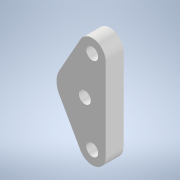
# Autodesk Inventor part: belt_tender_2
Saved by Autodesk Inventor 2020 (Build 240168000, 168)
## iProperties
Created: 2019-09-03
Part Number: belt_tender_2
Material: Generic
Document SubType Name: Modeling
Designer: psrob
Density: 1 g/cm^3
Appearance: Default
Author: psrob
Autodesk Inventor part; units mm, degrees
ref_plane "YZ Plane" through (0, 0, 0) normal (1, 0, 0) x (0, 1, 0)
ref_plane "XZ Plane" through (0, 0, 0) normal (0, 1, 0) x (-1, 0, 0)
ref_plane "XY Plane" through (0, 0, 0) normal (0, 0, 1) x (1, 0, 0)
sketch "Sketch1" plane through (0, 0, 0) normal (0, 0, 1) x (1, 0, 0)
  line L0 (0.625, 2.5) -> (2.625, 2.5) projected
  line L1 (4.125, 1) -> (2.625, 2.5) projected
  line L2 (4.125, 7) -> (4.125, 1) projected
  arc A0 (4.125, 7) -> (-0.0865, 8.1023) centre (1.875, 7) ccw projected
  line L3 (-3.6762, 1.7147) -> (-0.0865, 8.1023) projected
  arc A1 (-3.6762, 1.7147) -> (-3.6762, -1.7147) centre (-0.625, 0) ccw projected
  line L4 (-0.0865, -8.1023) -> (-3.6762, -1.7147) projected
  arc A2 (-0.0865, -8.1023) -> (4.125, -7) centre (1.875, -7) ccw projected
  line L5 (4.125, -1) -> (4.125, -7) projected
  line L6 (2.625, -2.5) -> (4.125, -1) projected
  line L7 (2.625, -2.5) -> (0.625, -2.5) projected
  arc A3 (0.625, 2.5) -> (0.625, -2.5) centre (0.625, 0) ccw projected
  circle A4 centre (1.875, 7) radius 1 projected
  circle A5 centre (1.875, -7) radius 1 projected
  circle A6 centre (0.625, 0) radius 1 projected
  line L8 (4.125, -1) -> (2.625, -2.5) projected
  line L9 (4.125, 1) -> (4.125, -1) projected
  line L10 (2.625, 2.5) -> (4.125, 1) projected
  line L11 (2.625, 2.5) -> (0.625, 2.5) projected
  arc A7 (0.625, 2.5) -> (0.625, -2.5) centre (0.625, 0) ccw projected
  line L12 (0.625, -2.5) -> (2.625, -2.5) projected
  point P0 (0, 0)
extrude "Extrusion1" add sketch "Sketch1" along normal blind 3
body "Solid1"
